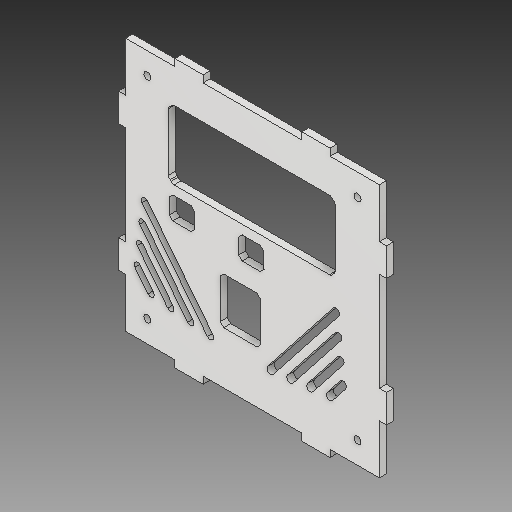
# Autodesk Inventor part: Face
Saved by Autodesk Inventor 2018.2 (Build 222227000, 227)
## iProperties
Created: 2018-04-16
Part Number: Face
Material: ABS Plastic
Document SubType Name: Modeling
Designer: Derek Fronek
Density: 1.06 g/cm^3
Appearance: Smooth - White
Author: Derek Fronek
Autodesk Inventor part; units mm, degrees
ref_plane "YZ Plane" through (0, 0, 0) normal (1, 0, 0) x (0, 1, 0)
ref_plane "XZ Plane" through (0, 0, 0) normal (0, 1, 0) x (-1, 0, 0)
ref_plane "XY Plane" through (0, 0, 0) normal (0, 0, 1) x (1, 0, 0)
sketch "Sketch1" plane through (0, 0, 0) normal (0, 0, 1) x (1, 0, 0)
  arc A0 (38.8267, -3.2916) -> (36.3322, -1.3274) centre (37.5794, -2.3095) ccw projected
  line L0 (38.8267, -3.2916) -> (9.3639, -40.7093) projected
  arc A1 (6.8694, -38.7451) -> (9.3639, -40.7093) centre (8.1167, -39.7272) ccw projected
  line L1 (6.8694, -38.7451) -> (36.3322, -1.3274) projected
  line L2 (39.8874, -12.209) -> (18.2813, -39.6486) projected
  arc A2 (15.7868, -37.6844) -> (18.2813, -39.6486) centre (17.0341, -38.6665) ccw projected
  line L3 (15.7868, -37.6844) -> (37.3928, -10.2448) projected
  arc A3 (39.8874, -12.209) -> (37.3928, -10.2448) centre (38.6401, -11.2269) ccw projected
  arc A4 (24.7042, -36.6238) -> (27.1987, -38.588) centre (25.9515, -37.6059) ccw projected
  line L4 (24.7042, -36.6238) -> (38.4535, -19.1622) projected
  arc A5 (40.948, -21.1264) -> (38.4535, -19.1622) centre (39.7008, -20.1443) ccw projected
  line L5 (40.948, -21.1264) -> (27.1987, -38.588) projected
  arc A6 (33.6216, -35.5631) -> (36.1161, -37.5273) centre (34.8689, -36.5452) ccw projected
  line L6 (33.6216, -35.5631) -> (39.5142, -28.0796) projected
  arc A7 (42.0087, -30.0438) -> (39.5142, -28.0796) centre (40.7614, -29.0617) ccw projected
  line L7 (42.0087, -30.0438) -> (36.1161, -37.5273) projected
  arc A8 (-50.4552, -28.0796) -> (-52.9497, -30.0438) centre (-51.7024, -29.0617) ccw projected
  line L8 (-50.4552, -28.0796) -> (-44.5626, -35.5631) projected
  arc A9 (-47.0571, -37.5273) -> (-44.5626, -35.5631) centre (-45.8099, -36.5452) ccw projected
  line L9 (-47.0571, -37.5273) -> (-52.9497, -30.0438) projected
  arc A10 (-49.3945, -19.1622) -> (-51.889, -21.1264) centre (-50.6418, -20.1443) ccw projected
  line L10 (-49.3945, -19.1622) -> (-35.6452, -36.6238) projected
  arc A11 (-38.1397, -38.588) -> (-35.6452, -36.6238) centre (-36.8925, -37.6059) ccw projected
  line L11 (-38.1397, -38.588) -> (-51.889, -21.1264) projected
  arc A12 (-48.3338, -10.2448) -> (-50.8284, -12.209) centre (-49.5811, -11.2269) ccw projected
  line L12 (-48.3338, -10.2448) -> (-26.7278, -37.6844) projected
  arc A13 (-29.2223, -39.6486) -> (-26.7278, -37.6844) centre (-27.9751, -38.6665) ccw projected
  line L13 (-29.2223, -39.6486) -> (-50.8284, -12.209) projected
  line L14 (-20.3049, -40.7093) -> (-49.7677, -3.2916) projected
  arc A14 (-47.2732, -1.3274) -> (-49.7677, -3.2916) centre (-48.5204, -2.3095) ccw projected
  line L15 (-47.2732, -1.3274) -> (-17.8104, -38.7451) projected
  arc A15 (-20.3049, -40.7093) -> (-17.8104, -38.7451) centre (-19.0577, -39.7272) ccw projected
  circle A16 centre (-47.3075, -47.3075) radius 1.6 projected
  circle A17 centre (47.3075, 47.3075) radius 1.6 projected
  circle A18 centre (-47.3075, 47.3075) radius 1.6 projected
  circle A19 centre (47.3075, -47.3075) radius 1.6 projected
  line L16 (-35.2867, 41.8525) -> (34.6517, 41.8525) projected
  arc A20 (35.9965, 41.1086) -> (34.6517, 41.8525) centre (34.6517, 40.265) ccw projected
  arc A21 (35.9965, 41.1086) -> (36.4386, 40.6665) centre (37.1825, 41.8525) ccw projected
  arc A22 (37.1825, 39.3217) -> (36.4386, 40.6665) centre (35.595, 39.3217) ccw projected
  line L17 (37.1825, 39.3217) -> (37.1825, 13.3833) projected
  arc A23 (36.4386, 12.0385) -> (37.1825, 13.3833) centre (35.595, 13.3833) ccw projected
  arc A24 (36.4386, 12.0385) -> (35.9965, 11.5964) centre (37.1825, 10.8525) ccw projected
  arc A25 (34.6517, 10.8525) -> (35.9965, 11.5964) centre (34.6517, 12.44) ccw projected
  line L18 (34.6517, 10.8525) -> (-35.2867, 10.8525) projected
  arc A26 (-36.6315, 11.5964) -> (-35.2867, 10.8525) centre (-35.2867, 12.44) ccw projected
  arc A27 (-36.6315, 11.5964) -> (-37.0736, 12.0385) centre (-37.8175, 10.8525) ccw projected
  arc A28 (-37.8175, 13.3833) -> (-37.0736, 12.0385) centre (-36.23, 13.3833) ccw projected
  line L19 (-37.8175, 13.3833) -> (-37.8175, 39.3217) projected
  arc A29 (-37.0736, 40.6665) -> (-37.8175, 39.3217) centre (-36.23, 39.3217) ccw projected
  arc A30 (-37.0736, 40.6665) -> (-36.6315, 41.1086) centre (-37.8175, 41.8525) ccw projected
  arc A31 (-35.2867, 41.8525) -> (-36.6315, 41.1086) centre (-35.2867, 40.265) ccw projected
  arc A32 (4.2545, -30.2586) -> (4.2545, -31.0524) centre (5.8045, -30.6555) ccw projected
  arc A33 (2.7142, -32.2555) -> (4.2545, -31.0524) centre (2.7142, -30.668) ccw projected
  line L20 (2.7142, -32.2555) -> (-13.608, -32.2555) projected
  arc A34 (-15.1955, -30.668) -> (-13.608, -32.2555) centre (-13.608, -30.668) ccw projected
  line L21 (-5.4705, -14.0555) -> (12.7295, -14.0555) construction
  line L22 (-14.551, -32.0455) -> (-14.551, -14.2655)
  line L23 (-12.9635, -12.678) -> (2.0225, -12.678)
  line L24 (3.61, -14.2655) -> (3.61, -32.0455)
  line L25 (2.0225, -33.633) -> (-12.9635, -33.633)
  line L26 (-14.551, -33.633) -> (3.61, -12.678) construction
  line L27 (-14.551, -12.678) -> (3.61, -33.633) construction
  line L28 (-14.551, -14.2655) -> (-12.9635, -12.678)
  line L29 (2.0225, -12.678) -> (3.61, -14.2655)
  line L30 (2.0225, -33.633) -> (3.61, -32.0455)
  line L31 (-14.551, -32.0455) -> (-12.9635, -33.633)
  line L32 (-4.6836, -3.4925) -> (3.5714, -3.4925)
  line L33 (5.1589, -1.905) -> (5.1589, 5.08)
  line L34 (3.5714, 6.6675) -> (-4.6836, 6.6675)
  line L35 (-6.2711, 5.08) -> (-6.2711, -1.905)
  line L36 (-6.2711, -3.4925) -> (5.1589, 6.6675) construction
  line L37 (5.1589, -3.4925) -> (-6.2711, 6.6675) construction
  line L38 (-6.2711, -3.4925) -> (1.9839, -3.4925) construction
  line L39 (-37.4655, -1.905) -> (-37.4655, 5.08)
  line L40 (-35.878, 6.6675) -> (-27.623, 6.6675)
  line L41 (-26.0355, 5.08) -> (-26.0355, -1.905)
  line L42 (-27.623, -3.4925) -> (-35.878, -3.4925)
  line L43 (-37.4655, -3.4925) -> (-26.0355, 6.6675) construction
  line L44 (-37.4655, 6.6675) -> (-26.0355, -3.4925) construction
  line L45 (-37.4655, 5.08) -> (-35.878, 6.6675)
  line L46 (-37.4655, -1.905) -> (-35.878, -3.4925)
  line L47 (-26.0355, -1.905) -> (-27.623, -3.4925)
  line L48 (-27.623, 6.6675) -> (-26.0355, 5.08)
  line L49 (-6.2711, 5.08) -> (-4.6836, 6.6675)
  line L50 (-4.6836, -3.4925) -> (-6.2711, -1.905)
  line L51 (3.5714, -3.4925) -> (5.1589, -1.905)
  line L52 (3.5714, 6.6675) -> (5.1589, 5.08)
  line L53 (34.925, 57.15) -> (34.925, 60.325)
  line L54 (34.925, 60.325) -> (22.225, 60.325)
  line L55 (22.225, 60.325) -> (22.225, 57.15)
  line L56 (-22.225, 57.15) -> (-22.225, 60.325)
  line L57 (-22.225, 60.325) -> (-34.925, 60.325)
  line L58 (-34.925, 60.325) -> (-34.925, 57.15)
  line L59 (-57.15, 57.15) -> (-34.925, 57.15)
  line L60 (-22.225, 57.15) -> (22.225, 57.15)
  line L61 (34.925, 57.15) -> (57.15, 57.15)
  line L62 (57.15, 0) -> (47.3075, 0)
  line L63 (-22.225, -57.15) -> (-22.225, -60.325)
  line L64 (-22.225, -60.325) -> (-34.925, -60.325)
  line L65 (-34.925, -60.325) -> (-34.925, -57.15)
  line L66 (22.225, -57.15) -> (22.225, -60.325)
  line L67 (22.225, -60.325) -> (34.925, -60.325)
  line L68 (34.925, -60.325) -> (34.925, -57.15)
  line L69 (-57.15, -57.15) -> (-34.925, -57.15)
  line L70 (-22.225, -57.15) -> (22.225, -57.15)
  line L71 (34.925, -57.15) -> (57.15, -57.15)
  line L72 (57.15, 34.925) -> (60.325, 34.925)
  line L73 (60.325, 34.925) -> (60.325, 22.225)
  line L74 (60.325, 22.225) -> (57.15, 22.225)
  line L75 (57.15, -57.15) -> (79.375, -57.15) construction
  line L76 (57.15, -34.925) -> (60.325, -34.925)
  line L77 (60.325, -34.925) -> (60.325, -22.225)
  line L78 (60.325, -22.225) -> (57.15, -22.225)
  line L79 (57.15, 57.15) -> (57.15, 34.925)
  line L80 (57.15, 22.225) -> (57.15, -22.225)
  line L81 (57.15, -34.925) -> (57.15, -57.15)
  line L82 (-57.15, 34.925) -> (-60.325, 34.925)
  line L83 (-60.325, 34.925) -> (-60.325, 22.225)
  line L84 (-60.325, 22.225) -> (-57.15, 22.225)
  line L85 (-57.15, -34.925) -> (-60.325, -34.925)
  line L86 (-60.325, -34.925) -> (-60.325, -22.225)
  line L87 (-60.325, -22.225) -> (-57.15, -22.225)
  line L88 (-57.15, 57.15) -> (-57.15, 34.925)
  line L89 (-57.15, 22.225) -> (-57.15, -22.225)
  line L90 (-57.15, -34.925) -> (-57.15, -57.15)
  point P0 (-5.4705, -23.1555)
  dimension "d1" = 20.955
  dimension "d2" = 18.161
  dimension "d3" = 1.5875
  dimension "d4" = 1.5875
  dimension "d5" = 1.5875
  dimension "d6" = 1.5875
  dimension "d7" = 1.5875
  dimension "d8" = 1.5875
  dimension "d9" = 1.5875
  dimension "d10" = 1.5875
  dimension "d11" = 11.43
  dimension "d12" = 0
  dimension "d13" = 10.16
  dimension "d14" = 11.43
  dimension "d15" = 1.5875
  dimension "d16" = 1.5875
  dimension "d17" = 1.5875
  dimension "d18" = 1.5875
  dimension "d19" = 1.5875
  dimension "d20" = 1.5875
  dimension "d21" = 1.5875
  dimension "d22" = 1.5875
  dimension "d23" = 1.5875
  dimension "d24" = 1.5875
  dimension "d25" = 1.5875
  dimension "d26" = 1.5875
  dimension "d27" = 1.5875
  dimension "d28" = 1.5875
  dimension "d29" = 1.5875
  dimension "d30" = 1.5875
  dimension "d36" = 3.175
  dimension "d38" = 12.7
  dimension "d39" = 3.175
  dimension "d40" = 12.7
  dimension "d41" = 3.175
  dimension "d42" = 12.7
  dimension "d43" = 22.225
  dimension "d44" = 3.175
  dimension "d45" = 12.7
  dimension "d46" = 22.225
  dimension "d48" = 12.7
  dimension "d49" = 3.175
  dimension "d50" = 12.7
  constraints: 140 end point, 25 point on line, 15 parallel, 13 horizontal, 7 collinear, 7 perpendicular, 2 midpoint, 2 vertical
  measures "d1" distance of L26.start L27.start
  measures "d2" distance of L27.start L26.end
  measures "d3" distance of L22.end L27.start
  measures "d4" distance of L23.start L27.start
  measures "d5" distance of L23.end L26.end
  measures "d6" distance of L24.start L26.end
  measures "d7" distance of L25.start L27.end
  measures "d8" distance of L24.end L27.end
  measures "d9" distance of L22.start L26.start
  measures "d10" distance of L25.end L26.start
  measures "d11" distance of L36.start L37.start
  measures "d12" distance between parallel lines of L32 L38
  measures "d13" distance of L36.end L37.start
  measures "d14" distance of L44.start L43.end
  measures "d15" distance of L39.end L44.start
  measures "d16" distance of L40.start L44.start
  measures "d17" distance of L39.start L43.start
  measures "d18" distance of L42.end L43.start
  measures "d19" distance of L41.end L44.end
  measures "d20" distance of L42.start L44.end
  measures "d21" distance of L40.end L43.end
  measures "d22" distance of L41.start L43.end
  measures "d23" distance of L35.start L37.end
  measures "d24" distance of L34.end L37.end
  measures "d25" distance of L32.start L36.start
  measures "d26" distance of L35.end L36.start
  measures "d27" distance of L32.end L37.start
  measures "d28" distance of L33.start L37.start
  measures "d29" distance of L34.start L36.end
  measures "d30" distance of L33.end L36.end
  measures "d36" distance of L53.end L53.start
  measures "d38" distance of L57.end L56.end
  measures "d39" distance of L56.end L56.start
  measures "d40" distance of L63.end L64.end
  measures "d41" distance of L63.start L63.end
  measures "d42" distance of L67.end L66.end
  measures "d43" distance of L61.end L72.start
  measures "d44" distance of L73.end L74.end
  measures "d45" distance of L72.end L73.end
  measures "d46" distance of L71.end L76.start
  measures "d48" distance of L77.end L76.end
  measures "d49" distance of L84.end L83.end
  measures "d50" distance of L85.end L86.end
extrude "Extrusion1" add sketch "Sketch1" along normal blind 3.175
equation "\"d4\" = d3"
equation "\"d5\" = d3"
equation "\"d6\" = d5"
equation "\"d7\" = d3"
equation "\"d8\" = d7"
equation "\"d9\" = d3"
equation "\"d10\" = d9"
equation "\"d16\" = d15"
equation "\"d18\" = d17"
equation "\"d19\" = d17"
equation "\"d20\" = d19"
equation "\"d21\" = d17"
equation "\"d22\" = d21"
equation "\"d23\" = d17"
equation "\"d24\" = d23"
equation "\"d25\" = d17"
equation "\"d26\" = d25"
equation "\"d27\" = d17"
equation "\"d28\" = d27"
equation "\"d29\" = d17"
equation "\"d30\" = d29"
body "Solid1"
